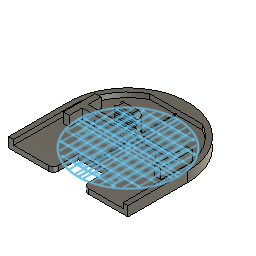
shadowmask_wafer_cleaver (Autodesk Fusion 360 design; units mm, degrees)
Autodesk Fusion 360 part; units mm, degrees
note: some values were not read from the file. Set by a fixed rule: which sketch regions a step uses.
(part 1 of 3)
sketch "wafer_condensed" plane through (0, 0, 0) normal (0, 0, 1) x (1, 0, 0)
  line L0 (3.9115, 15.9115) -> (2, 15.9115)
  line L1 (-4.0885, 2) -> (-4.0885, 3.9115)
  line L2 (-38.9115, 4.0885) -> (-39.0885, 4.0885)
  line L3 (-24.9115, 3.9115) -> (-18.0885, 3.9115)
  line L4 (-31.9115, 3.9115) -> (-25.0885, 3.9115)
  line L5 (-11.0885, 3.9115) -> (-10.9115, 3.9115)
  line L6 (-25.0885, 4.0885) -> (-25.0885, 3.9115)
  line L7 (-39.0885, 3.9115) -> (-38.9115, 3.9115)
  line L8 (-25.0885, 3.9115) -> (-31.9115, 3.9115)
  line L9 (-3.9115, 3.9115) -> (-2, 3.9115)
  line L10 (-32.0885, 3.9115) -> (-31.9115, 3.9115)
  line L11 (-10.9115, 3.9115) -> (-4.0885, 3.9115)
  line L12 (-25.0885, 3.9115) -> (-24.9115, 3.9115)
  line L13 (-31.9115, 3.9115) -> (-31.9115, 4.0885)
  line L14 (-4.0885, 3.9115) -> (-3.9115, 3.9115)
  line L15 (-3.9115, 3.9115) -> (-3.9115, 2)
  line L16 (-2, 3.9115) -> (-3.9115, 3.9115)
  line L17 (-32.0885, 3.9115) -> (-38.9115, 3.9115)
  line L18 (-32.0885, 4.0885) -> (-32.0885, 3.9115)
  line L19 (-10.9115, 3.9115) -> (-10.9115, 2)
  line L20 (-24.9115, 3.9115) -> (-24.9115, 4.0885)
  line L21 (-4.0885, 3.9115) -> (-10.9115, 3.9115)
  line L22 (-18.0885, 3.9115) -> (-17.9115, 3.9115)
  line L23 (-10.9115, 2) -> (-11.0885, 2)
  line L24 (-17.9115, 3.9115) -> (-11.0885, 3.9115)
  line L25 (-38.9115, 3.9115) -> (-38.9115, 4.0885)
  line L26 (-24.9115, 4.0885) -> (-25.0885, 4.0885)
  line L27 (-3.9115, 2) -> (-4.0885, 2)
  line L28 (-11.0885, 2) -> (-11.0885, 3.9115)
  line L29 (-39.0885, 4.0885) -> (-39.0885, 3.9115)
  line L30 (-18.0885, 3.9115) -> (-24.9115, 3.9115)
  line L31 (-38.9115, 3.9115) -> (-32.0885, 3.9115)
  line L32 (-45.9115, 2) -> (-46.0885, 2)
  line L33 (-25.0885, 3.9115) -> (-31.9115, 3.9115)
  line L34 (-45.9115, 3.9115) -> (-45.9115, 2)
  line L35 (-39.0885, 3.9115) -> (-45.9115, 3.9115)
  line L36 (-32.0885, 2) -> (-32.0885, 3.9115)
  line L37 (-18.0885, 2) -> (-18.0885, 3.9115)
  line L38 (-18.0885, 3.9115) -> (-24.9115, 3.9115)
  line L39 (-39.0885, 2) -> (-39.0885, 3.9115)
  line L40 (-38.9115, 2) -> (-39.0885, 2)
  line L41 (-31.9115, 2) -> (-32.0885, 2)
  line L42 (-10.9115, -46.7226) -> (-11.0885, -46.7226)
  line L43 (-24.9115, 3.9115) -> (-24.9115, 2)
  line L44 (-11.0885, -46.7226) -> (-11.0885, -40.0885)
  line L45 (-32.0885, 3.9115) -> (-38.9115, 3.9115)
  line L46 (-17.9115, 2) -> (-18.0885, 2)
  line L47 (-11.0885, -40.0885) -> (-17.9115, -40.0885)
  line L48 (-4.0885, -47.833) -> (-4.0885, -40.0885)
  line L49 (-24.9115, 2) -> (-25.0885, 2)
  line L50 (-17.9115, 3.9115) -> (-17.9115, 2)
  line L51 (-11.0885, 3.9115) -> (-17.9115, 3.9115)
  line L52 (-10.9115, -40.0885) -> (-10.9115, -46.7226)
  line L53 (-25.0885, 2) -> (-25.0885, 3.9115)
  line L54 (-4.0885, -40.0885) -> (-10.9115, -40.0885)
  line L55 (-31.9115, 3.9115) -> (-31.9115, 2)
  line L56 (-38.9115, 3.9115) -> (-38.9115, 2)
  line L57 (-17.9115, 39.9115) -> (-17.9115, 28.0885)
  line L58 (-11.0885, 27.9115) -> (-17.9115, 27.9115)
  line L59 (-3.9115, 28.0885) -> (-4.0885, 28.0885)
  line L60 (-24.9115, 39.9115) -> (-24.9115, 28.0885)
  line L61 (-38.9115, 27.9115) -> (-38.9115, 16.0885)
  line L62 (-4.0885, 16.0885) -> (-4.0885, 27.9115)
  line L63 (-17.9115, 16.0885) -> (-11.0885, 16.0885)
  line L64 (-18.0885, 28.0885) -> (-18.0885, 39.9115)
  line L65 (-18.0885, 16.0885) -> (-18.0885, 27.9115)
  line L66 (-38.9872, 27.9821) -> (-38.9872, 27.9115)
  line L67 (-17.9115, 16.0885) -> (-18.0885, 16.0885)
  line L68 (-32.0885, 16.0885) -> (-31.9115, 16.0885)
  line L69 (-32.0885, 16.0885) -> (-32.0885, 27.9115)
  line L70 (-18.0885, 27.9115) -> (-17.9115, 27.9115)
  line L71 (-31.9115, 16.0885) -> (-32.0885, 16.0885)
  line L72 (-32.0885, 28.0885) -> (-32.0885, 27.9115)
  line L73 (-3.9115, 16.0885) -> (-4.0885, 16.0885)
  line L74 (-25.0885, 16.0885) -> (-25.0885, 27.9115)
  line L75 (-11.0885, 28.0885) -> (-11.0885, 27.9115)
  line L76 (-31.9115, 27.9115) -> (-31.9115, 16.0885)
  line L77 (-11.0885, 15.9115) -> (-17.9115, 15.9115)
  line L78 (-10.9115, 15.9115) -> (-10.9115, 16.0885)
  line L79 (-25.0885, 28.0885) -> (-25.0885, 27.9115)
  line L80 (-2, 27.9115) -> (-3.9115, 27.9115)
  line L81 (-24.9115, 16.0885) -> (-25.0885, 16.0885)
  line L82 (-11.0885, 15.9115) -> (-10.9115, 15.9115)
  line L83 (-17.9115, 28.0885) -> (-18.0885, 28.0885)
  line L84 (-3.9115, 27.9115) -> (-2, 27.9115)
  line L85 (-10.9115, 27.9115) -> (-4.0885, 27.9115)
  line L86 (-10.9115, 28.0885) -> (-4.0885, 28.0885)
  line L87 (-25.0885, 27.9115) -> (-31.9115, 27.9115)
  line L88 (-25.0885, 15.9115) -> (-24.9115, 15.9115)
  line L89 (-2, 16.0885) -> (-2, 15.9115)
  line L90 (-31.9115, 27.9115) -> (-31.9115, 28.0885)
  line L91 (-11.0885, 27.9115) -> (-17.9115, 27.9115)
  line L92 (-18.0885, 28.0885) -> (-17.9115, 28.0885)
  line L93 (-17.9115, 27.9115) -> (-17.9115, 28.0885)
  line L94 (-24.9115, 28.0885) -> (-18.0885, 28.0885)
  line L95 (-4.0885, 27.9115) -> (-10.9115, 27.9115)
  line L96 (-4.0885, 4.0885) -> (-3.9115, 4.0885)
  line L97 (-10.9115, 28.0885) -> (-11.0885, 28.0885)
  line L98 (-17.9115, 28.0885) -> (-18.0885, 28.0885)
  line L99 (-25.0885, 4.0885) -> (-24.9115, 4.0885)
  line L100 (-31.9115, 15.9115) -> (-31.9115, 16.0885)
  line L101 (-25.0885, 15.9115) -> (-31.9115, 15.9115)
  line L102 (-24.9115, 15.9115) -> (-18.0885, 15.9115)
  line L103 (-31.9115, 28.0885) -> (-32.0885, 28.0885)
  line L104 (-4.0885, 16.0885) -> (-4.0885, 15.9115)
  line L105 (-11.0885, 4.0885) -> (-10.9115, 4.0885)
  line L106 (-18.0885, 16.0885) -> (-17.9115, 16.0885)
  line L107 (-25.0885, 4.0885) -> (-25.0885, 15.9115)
  line L108 (-4.0885, 27.9115) -> (-3.9115, 27.9115)
  line L109 (-17.9115, 27.9115) -> (-11.0885, 27.9115)
  line L110 (-25.0885, 27.9115) -> (-31.9115, 27.9115)
  line L111 (-11.0885, 16.0885) -> (-11.0885, 27.9115)
  line L112 (-17.9115, 15.9115) -> (-17.9115, 16.0885)
  line L113 (-4.0885, 27.9115) -> (-10.9115, 27.9115)
  line L114 (-11.0885, 27.9115) -> (-10.9115, 27.9115)
  line L115 (-32.0885, 4.0885) -> (-31.9115, 4.0885)
  line L116 (-18.0885, 27.9115) -> (-24.9115, 27.9115)
  line L117 (-4.0885, 28.0885) -> (-4.0885, 27.9115)
  line L118 (-24.9115, 4.0885) -> (-18.0885, 4.0885)
  line L119 (-11.0885, 28.0885) -> (-10.9115, 28.0885)
  line L120 (-2, 4.0885) -> (-2, 3.9115)
  line L121 (-2, 15.9115) -> (-3.9115, 15.9115)
  line L122 (-11.0885, 16.0885) -> (-10.9115, 16.0885)
  line L123 (-10.9115, 27.9115) -> (-10.9115, 28.0885)
  line L124 (-4.0885, 4.0885) -> (-4.0885, 15.9115)
  line L125 (-18.0885, 28.0885) -> (-18.0885, 27.9115)
  line L126 (-4.0885, 15.9115) -> (-10.9115, 15.9115)
  line L127 (-2, 15.9115) -> (-3.9115, 15.9115)
  line L128 (-18.0885, 4.0885) -> (-18.0885, 15.9115)
  line L129 (-17.9115, 15.9115) -> (-17.9115, 4.0885)
  line L130 (-17.9115, 4.0885) -> (-11.0885, 4.0885)
  line L131 (-11.0885, 15.9115) -> (-17.9115, 15.9115)
  line L132 (-4.0885, 15.9115) -> (-10.9115, 15.9115)
  line L133 (-3.9115, 4.0885) -> (-2, 4.0885)
  line L134 (-10.9115, 4.0885) -> (-11.0885, 4.0885)
  line L135 (-3.9115, 15.9115) -> (-3.9115, 4.0885)
  line L136 (-25.0885, 16.0885) -> (-24.9115, 16.0885)
  line L137 (-25.0885, 15.9115) -> (-31.9115, 15.9115)
  line L138 (-18.0885, 15.9115) -> (-24.9115, 15.9115)
  line L139 (-38.9115, 27.9821) -> (-38.9872, 27.9821)
  line L140 (-3.9115, 15.9115) -> (-2, 15.9115)
  line L141 (-17.9115, 28.0885) -> (-11.0885, 28.0885)
  line L142 (-4.0885, 15.9115) -> (-3.9115, 15.9115)
  line L143 (-24.9115, 15.9115) -> (-24.9115, 4.0885)
  line L144 (-24.9115, 16.0885) -> (-18.0885, 16.0885)
  line L145 (-3.9115, 16.0885) -> (-2, 16.0885)
  line L146 (-17.9115, 27.9115) -> (-17.9115, 16.0885)
  line L147 (-18.0885, 4.0885) -> (-17.9115, 4.0885)
  line L148 (-4.0885, 16.0885) -> (-3.9115, 16.0885)
  line L149 (-10.9115, 16.0885) -> (-4.0885, 16.0885)
  line L150 (-24.9115, 16.0885) -> (-25.0885, 16.0885)
  line L151 (-32.0885, 27.9115) -> (-31.9115, 27.9115)
  line L152 (-10.9115, 15.9115) -> (-4.0885, 15.9115)
  line L153 (-10.9115, 15.9115) -> (-10.9115, 4.0885)
  line L154 (-32.0885, 4.0885) -> (-32.0885, 15.9115)
  line L155 (-3.9115, 27.9115) -> (-3.9115, 16.0885)
  line L156 (-25.0885, 16.0885) -> (-25.0885, 15.9115)
  line L157 (-32.0885, 15.9115) -> (-31.9115, 15.9115)
  line L158 (-32.0885, 27.9115) -> (-38.9115, 27.9115)
  line L159 (-31.9115, 16.0885) -> (-25.0885, 16.0885)
  line L160 (-32.0885, 15.9115) -> (-38.9115, 15.9115)
  line L161 (-31.9115, 16.0885) -> (-32.0885, 16.0885)
  line L162 (-38.9115, 27.9115) -> (-38.9115, 27.9821)
  line L163 (-18.0885, 27.9115) -> (-24.9115, 27.9115)
  line L164 (-24.9115, 27.9115) -> (-24.9115, 28.0885)
  line L165 (-18.0885, 39.9115) -> (-24.9115, 39.9115)
  line L166 (-4.0885, 28.0885) -> (-3.9115, 28.0885)
  line L167 (-17.9115, 16.0885) -> (-18.0885, 16.0885)
  line L168 (-24.9115, 15.9115) -> (-24.9115, 16.0885)
  line L169 (-24.9115, 27.9115) -> (-18.0885, 27.9115)
  line L170 (-10.9115, 16.0885) -> (-11.0885, 16.0885)
  line L171 (-31.9115, 4.0885) -> (-32.0885, 4.0885)
  line L172 (-2, 28.0885) -> (-2, 27.9115)
  line L173 (-10.9115, 4.0885) -> (-4.0885, 4.0885)
  line L174 (-2, 27.9115) -> (-3.9115, 27.9115)
  line L175 (-24.9115, 28.0885) -> (-25.0885, 28.0885)
  line L176 (-32.0885, 27.9115) -> (-38.9115, 27.9115)
  line L177 (-11.0885, 16.0885) -> (-11.0885, 15.9115)
  line L178 (-3.9115, 4.0885) -> (-4.0885, 4.0885)
  line L179 (-32.0885, 16.0885) -> (-32.0885, 15.9115)
  line L180 (-17.9115, 4.0885) -> (-18.0885, 4.0885)
  line L181 (-31.9115, 4.0885) -> (-25.0885, 4.0885)
  line L182 (-25.0885, 27.9115) -> (-24.9115, 27.9115)
  line L183 (-3.9115, 16.0885) -> (-4.0885, 16.0885)
  line L184 (-38.9115, 15.9115) -> (-38.9115, 4.0885)
  line L185 (-24.9115, 27.9115) -> (-24.9115, 16.0885)
  line L186 (-3.9115, 15.9115) -> (-3.9115, 16.0885)
  line L187 (-31.9115, 15.9115) -> (-31.9115, 4.0885)
  line L188 (-10.9115, 16.0885) -> (-11.0885, 16.0885)
  line L189 (-10.9115, 27.9115) -> (-10.9115, 16.0885)
  line L190 (-31.9115, 15.9115) -> (-25.0885, 15.9115)
  line L191 (-38.9115, 16.0885) -> (-32.0885, 16.0885)
  line L192 (-3.9115, 27.9115) -> (-3.9115, 28.0885)
  line L193 (-18.0885, 15.9115) -> (-17.9115, 15.9115)
  line L194 (-31.9115, 27.9115) -> (-25.0885, 27.9115)
  line L195 (-3.9115, 28.0885) -> (-2, 28.0885)
  line L196 (-18.0885, 15.9115) -> (-24.9115, 15.9115)
  line L197 (-24.9115, 4.0885) -> (-25.0885, 4.0885)
  line L198 (-38.9872, 27.9115) -> (-38.9115, 27.9115)
  line L199 (-11.0885, 4.0885) -> (-11.0885, 15.9115)
  line L200 (-38.9115, 4.0885) -> (-32.0885, 4.0885)
  line L201 (-18.0885, 16.0885) -> (-18.0885, 15.9115)
  line L202 (-17.9115, 15.9115) -> (-11.0885, 15.9115)
  line L203 (-38.9115, 27.9115) -> (-32.0885, 27.9115)
  line L204 (-17.9115, 3.9115) -> (-17.9115, 4.0885)
  line L205 (-4.0885, 4.0885) -> (-4.0885, 3.9115)
  line L206 (-3.9115, 4.0885) -> (-4.0885, 4.0885)
  line L207 (-17.9115, 4.0885) -> (-18.0885, 4.0885)
  line L208 (-11.0885, 3.9115) -> (-17.9115, 3.9115)
  line L209 (-3.9115, 3.9115) -> (-3.9115, 4.0885)
  line L210 (-18.0885, 4.0885) -> (-18.0885, 3.9115)
  line L211 (-2, 3.9115) -> (-3.9115, 3.9115)
  line L212 (-11.0885, 4.0885) -> (-11.0885, 3.9115)
  line L213 (-4.0885, 3.9115) -> (-10.9115, 3.9115)
  line L214 (-10.9115, 3.9115) -> (-10.9115, 4.0885)
  line L215 (-10.9115, 4.0885) -> (-11.0885, 4.0885)
  line L216 (-10.9115, 39.9115) -> (-4.0885, 39.9115)
  line L217 (-11.0885, 28.0885) -> (-11.0885, 39.9115)
  line L218 (-10.9115, 39.9115) -> (-10.9115, 28.0885)
  line L219 (-4.0885, 39.9115) -> (-10.9115, 39.9115)
  line L220 (-3.9115, 28.0885) -> (-4.0885, 28.0885)
  line L221 (-10.9115, 28.0885) -> (-11.0885, 28.0885)
  line L222 (-4.0885, 28.0885) -> (-4.0885, 39.9115)
  line L223 (-11.0885, 39.9115) -> (-17.9115, 39.9115)
  line L224 (-3.9115, 39.9115) -> (-2, 39.9115)
  line L225 (-2, 39.9115) -> (-3.9115, 39.9115)
  line L226 (-4.0885, 39.9115) -> (-3.9115, 39.9115)
  line L227 (-3.9115, 39.9115) -> (-3.9115, 28.0885)
  line L228 (18.0885, 2) -> (17.9115, 2)
  line L229 (3.9115, 40.0885) -> (3.9115, 39.9115)
  line L230 (-46.0885, 3.9115) -> (-47.833, 3.9115)
  line L231 (17.9115, 3.9115) -> (11.0885, 3.9115)
  line L232 (39.0885, 15.9115) -> (39.0885, 16.0885)
  line L233 (18.0885, 40.0885) -> (24.9115, 40.0885)
  line L234 (24.9115, 39.9115) -> (25.0885, 39.9115)
  line L235 (3.9115, 39.9115) -> (2, 39.9115)
  line L236 (-45.9115, 13.7113) -> (-45.9115, 4.0885)
  line L237 (31.9115, 3.9115) -> (25.0885, 3.9115)
  line L238 (46.0885, 3.9115) -> (46.0885, 4.0885)
  line L239 (-25.0885, 39.9115) -> (-26.533, 39.9115)
  line L240 (25.0885, 3.9115) -> (25.0885, 2)
  line L241 (38.9115, 3.9115) -> (32.0885, 3.9115)
  line L242 (38.9115, 2) -> (38.9115, 3.9115)
  line L243 (-25.0885, 40.0885) -> (-25.0885, 39.9115)
  line L244 (46.0885, 4.0885) -> (45.9115, 4.0885)
  line L245 (31.9115, 35.7771) -> (32.0885, 35.7771)
  line L246 (-39.0885, 16.0885) -> (-39.0885, 27.9821)
  line L247 (4.0885, 40.0885) -> (10.9115, 40.0885)
  line L248 (-38.9115, 15.9115) -> (-38.9115, 16.0885)
  line L249 (17.9115, 2) -> (17.9115, 3.9115)
  line L250 (2, 39.9115) -> (2, 40.0885)
  line L251 (2, 40.0885) -> (3.9115, 40.0885)
  line L252 (-24.9115, 39.9115) -> (-24.9115, 40.0885)
  line L253 (38.9872, 27.9821) -> (39.0885, 27.9821)
  line L254 (24.9115, 40.0885) -> (24.9115, 40.9756)
  line L255 (-46.0885, 4.0885) -> (-46.0885, 3.9115)
  line L256 (39.0885, 27.9821) -> (39.0885, 16.0885)
  line L257 (-38.9872, 28.0885) -> (-32.0885, 28.0885)
  line L258 (11.0885, 3.9115) -> (11.0885, 2)
  line L259 (4.0885, 40.0885) -> (3.9115, 40.0885)
  line L260 (4.0885, 39.9115) -> (4.0885, 40.0885)
  line L261 (45.9115, 2) -> (45.9115, 3.9115)
  line L262 (-46.0885, 3.9115) -> (-45.9115, 3.9115)
  line L263 (25.0885, 40.0885) -> (26.533, 40.0885)
  line L264 (-39.0885, 4.0885) -> (-39.0885, 15.9115)
  line L265 (38.9872, 28.0885) -> (38.9872, 27.9821)
  line L266 (47.833, 3.9115) -> (46.0885, 3.9115)
  line L267 (32.0885, 3.9115) -> (32.0885, 2)
  line L268 (11.0885, 46.7226) -> (11.0885, 40.0885)
  line L269 (17.9115, 44.4972) -> (18.0885, 44.4972)
  line L270 (-46.0885, 2) -> (-46.0885, 3.9115)
  line L271 (4.0885, 3.9115) -> (4.0885, 2)
  line L272 (31.9115, 28.0885) -> (31.9115, 35.7771)
  line L273 (10.9115, 39.9115) -> (4.0885, 39.9115)
  line L274 (-45.2548, 15.9115) -> (-45.2548, 16.0885)
  line L275 (24.9115, 3.9115) -> (18.0885, 3.9115)
  line L276 (-39.0885, 15.9115) -> (-45.2548, 15.9115)
  line L277 (-47.833, 3.9115) -> (-47.833, 4.0885)
  line L278 (-45.9115, 4.0885) -> (-46.0885, 4.0885)
  line L279 (10.9115, 3.9115) -> (4.0885, 3.9115)
  line L280 (26.533, 40.0885) -> (26.533, 39.9115)
  line L281 (31.9115, 2) -> (31.9115, 3.9115)
  line L282 (-25.0885, 28.0885) -> (-25.0885, 39.9115)
  line L283 (26.533, 39.9115) -> (25.0885, 39.9115)
  line L284 (-39.0885, 15.9115) -> (-38.9115, 15.9115)
  line L285 (25.0885, 40.9756) -> (25.0885, 40.0885)
  line L286 (32.0885, 2) -> (31.9115, 2)
  line L287 (45.9115, 3.9115) -> (39.0885, 3.9115)
  line L288 (11.0885, 2) -> (10.9115, 2)
  line L289 (25.0885, 39.9115) -> (25.0885, 28.0885)
  line L290 (39.0885, 4.0885) -> (45.9115, 4.0885)
  line L291 (25.0885, 40.0885) -> (24.9115, 40.0885)
  line L292 (-24.9115, 40.0885) -> (-25.0885, 40.0885)
  line L293 (18.0885, 3.9115) -> (18.0885, 2)
  line L294 (4.0885, 2) -> (3.9115, 2)
  line L295 (32.0885, 28.0885) -> (38.9872, 28.0885)
  line L296 (45.9115, 13.7113) -> (46.0885, 13.7113)
  line L297 (32.0885, 35.7771) -> (32.0885, 28.0885)
  line L298 (3.9115, 40.0885) -> (3.9115, 47.833)
  line L299 (24.9115, 2) -> (24.9115, 3.9115)
  line L300 (-47.833, 4.0885) -> (-46.0885, 4.0885)
  line L301 (39.0885, 15.9115) -> (39.0885, 4.0885)
  line L302 (46.0885, 2) -> (45.9115, 2)
  line L303 (45.9115, 4.0885) -> (45.9115, 13.7113)
  line L304 (38.9115, 15.9115) -> (39.0885, 15.9115)
  line L305 (39.0885, 2) -> (38.9115, 2)
  line L306 (3.9115, 47.833) -> (4.0885, 47.833)
  line L307 (46.0885, 3.9115) -> (46.0885, 2)
  line L308 (-39.0885, 16.0885) -> (-39.0885, 15.9115)
  line L309 (47.833, 4.0885) -> (47.833, 3.9115)
  line L310 (25.0885, 2) -> (24.9115, 2)
  line L311 (10.9115, 2) -> (10.9115, 3.9115)
  line L312 (11.0885, 40.0885) -> (17.9115, 40.0885)
  line L313 (-45.9115, 4.0885) -> (-39.0885, 4.0885)
  line L314 (45.2548, 16.0885) -> (45.2548, 15.9115)
  line L315 (-32.0885, 35.7771) -> (-31.9115, 35.7771)
  line L316 (25.0885, 39.9115) -> (25.0885, 40.0885)
  line L317 (46.0885, 13.7113) -> (46.0885, 4.0885)
  line L318 (10.9115, 46.7226) -> (11.0885, 46.7226)
  line L319 (24.9115, 40.9756) -> (25.0885, 40.9756)
  line L320 (18.0885, 44.4972) -> (18.0885, 40.0885)
  line L321 (-25.0885, 39.9115) -> (-24.9115, 39.9115)
  line L322 (-31.9115, 35.7771) -> (-31.9115, 28.0885)
  line L323 (39.0885, 3.9115) -> (39.0885, 2)
  line L324 (-46.0885, 4.0885) -> (-46.0885, 13.7113)
  line L325 (-46.0885, 13.7113) -> (-45.9115, 13.7113)
  line L326 (24.9115, 40.0885) -> (24.9115, 39.9115)
  line L327 (45.9115, 3.9115) -> (46.0885, 3.9115)
  line L328 (25.0885, 28.0885) -> (31.9115, 28.0885)
  line L329 (45.9115, 4.0885) -> (45.9115, 3.9115)
  line L330 (39.0885, 16.0885) -> (45.2548, 16.0885)
  line L331 (38.9115, 16.0885) -> (38.9115, 15.9115)
  line L332 (10.9115, 40.0885) -> (10.9115, 39.9115)
  line L333 (-32.0885, 28.0885) -> (-32.0885, 35.7771)
  line L334 (-39.0885, 27.9821) -> (-38.9872, 27.9821)
  line L335 (10.9115, 40.0885) -> (10.9115, 46.7226)
  line L336 (-45.9115, 3.9115) -> (-45.9115, 4.0885)
  line L337 (-45.2548, 16.0885) -> (-39.0885, 16.0885)
  line L338 (46.0885, 4.0885) -> (47.833, 4.0885)
  line L339 (17.9115, 40.0885) -> (17.9115, 44.4972)
  line L340 (-38.9872, 27.9821) -> (-38.9872, 28.0885)
  line L341 (-31.9115, 28.0885) -> (-25.0885, 28.0885)
  line L342 (45.2548, 15.9115) -> (39.0885, 15.9115)
  line L343 (39.0885, 16.0885) -> (38.9115, 16.0885)
  line L344 (4.0885, 47.833) -> (4.0885, 40.0885)
  line L345 (-38.9115, 16.0885) -> (-39.0885, 16.0885)
  line L346 (-17.9115, 39.9115) -> (-17.9115, 40.0885)
  line L347 (-18.0885, 44.4972) -> (-17.9115, 44.4972)
  line L348 (-25.0885, 40.9756) -> (-24.9115, 40.9756)
  line L349 (-11.0885, 40.0885) -> (-11.0885, 46.7226)
  line L350 (-18.0885, 40.0885) -> (-18.0885, 39.9115)
  line L351 (-11.0885, 39.9115) -> (-17.9115, 39.9115)
  line L352 (-11.0885, 40.0885) -> (-11.0885, 39.9115)
  line L353 (-18.0885, 39.9115) -> (-17.9115, 39.9115)
  line L354 (-26.533, 39.9115) -> (-26.533, 40.0885)
  line L355 (-26.533, 40.0885) -> (-25.0885, 40.0885)
  line L356 (-4.0885, 40.0885) -> (-4.0885, 47.833)
  line L357 (-3.9115, 39.9115) -> (-3.9115, 40.0885)
  line L358 (-24.9115, 40.0885) -> (-18.0885, 40.0885)
  line L359 (-3.9115, 40.0885) -> (-4.0885, 40.0885)
  line L360 (-17.9115, 40.0885) -> (-18.0885, 40.0885)
  line L361 (-17.9115, 40.0885) -> (-11.0885, 40.0885)
  line L362 (-4.0885, 47.833) -> (-3.9115, 47.833)
  line L363 (-10.9115, 40.0885) -> (-4.0885, 40.0885)
  line L364 (-3.9115, 40.0885) -> (-2, 40.0885)
  line L365 (-17.9115, 44.4972) -> (-17.9115, 40.0885)
  line L366 (-25.0885, 40.0885) -> (-25.0885, 40.9756)
  line L367 (-11.0885, 46.7226) -> (-10.9115, 46.7226)
  line L368 (-2, 40.0885) -> (-2, 39.9115)
  line L369 (-10.9115, 46.7226) -> (-10.9115, 40.0885)
  line L370 (-4.0885, 40.0885) -> (-4.0885, 39.9115)
  line L371 (-24.9115, 40.9756) -> (-24.9115, 40.0885)
  line L372 (-2, 39.9115) -> (-3.9115, 39.9115)
  line L373 (-10.9115, 40.0885) -> (-11.0885, 40.0885)
  line L374 (-4.0885, 39.9115) -> (-10.9115, 39.9115)
  line L375 (-18.0885, 40.0885) -> (-18.0885, 44.4972)
  line L376 (-10.9115, 39.9115) -> (-10.9115, 40.0885)
  line L377 (-3.9115, 47.833) -> (-3.9115, 40.0885)
  line L378 (-11.0885, 39.9115) -> (-10.9115, 39.9115)
  line L379 (-17.9115, 39.9115) -> (-11.0885, 39.9115)
  line L380 (10.9115, -15.9115) -> (4.0885, -15.9115)
  line L381 (4.0885, 4.0885) -> (3.9115, 4.0885)
  line L382 (47.833, -3.9115) -> (47.833, -4.0885)
  line L383 (47.833, -4.0885) -> (46.0885, -4.0885)
  line L384 (4.0885, 3.9115) -> (10.9115, 3.9115)
  line L385 (10.9115, 3.9115) -> (11.0885, 3.9115)
  line L386 (17.9115, 3.9115) -> (18.0885, 3.9115)
  line L387 (18.0885, 4.0885) -> (17.9115, 4.0885)
  line L388 (4.0885, -15.9115) -> (3.9115, -15.9115)
  line L389 (11.0885, 3.9115) -> (17.9115, 3.9115)
  line L390 (4.0885, -15.9115) -> (10.9115, -15.9115)
  line L391 (24.9115, -40.9756) -> (24.9115, -40.0885)
  line L392 (38.9115, -16.0885) -> (39.0885, -16.0885)
  line L393 (32.0885, 4.0885) -> (31.9115, 4.0885)
  line L394 (11.0885, 4.0885) -> (17.9115, 4.0885)
  line L395 (18.0885, -15.9115) -> (17.9115, -15.9115)
  line L396 (25.0885, 4.0885) -> (31.9115, 4.0885)
  line L397 (3.9115, 4.0885) -> (4.0885, 4.0885)
  line L398 (11.0885, -40.0885) -> (11.0885, -46.7226)
  line L399 (26.533, -39.9115) -> (26.533, -40.0885)
  line L400 (25.0885, -39.9115) -> (26.533, -39.9115)
  line L401 (11.0885, -46.7226) -> (10.9115, -46.7226)
  line L402 (39.0885, -15.9115) -> (45.2548, -15.9115)
  line L403 (45.2548, -15.9115) -> (45.2548, -16.0885)
  line L404 (45.9115, -4.0885) -> (39.0885, -4.0885)
  line L405 (39.0885, -16.0885) -> (39.0885, -27.9821)
  line L406 (4.0885, -40.0885) -> (4.0885, -47.833)
  line L407 (45.2548, -16.0885) -> (39.0885, -16.0885)
  line L408 (38.9115, 3.9115) -> (39.0885, 3.9115)
  line L409 (39.0885, -15.9115) -> (38.9115, -15.9115)
  line L410 (32.0885, -35.7771) -> (31.9115, -35.7771)
  line L411 (10.9115, -40.0885) -> (4.0885, -40.0885)
  line L412 (24.9115, 3.9115) -> (25.0885, 3.9115)
  line L413 (10.9115, -46.7226) -> (10.9115, -40.0885)
  line L414 (38.9872, -28.0885) -> (32.0885, -28.0885)
  line L415 (25.0885, -28.0885) -> (25.0885, -39.9115)
  line L416 (31.9115, -28.0885) -> (25.0885, -28.0885)
  line L417 (32.0885, -28.0885) -> (32.0885, -35.7771)
  line L418 (18.0885, 15.9115) -> (18.0885, 4.0885)
  line L419 (32.0885, 15.9115) -> (32.0885, 4.0885)
  line L420 (25.0885, -40.0885) -> (25.0885, -39.9115)
  line L421 (3.9115, 3.9115) -> (2, 3.9115)
  line L422 (18.0885, 3.9115) -> (24.9115, 3.9115)
  line L423 (18.0885, -44.4972) -> (17.9115, -44.4972)
  line L424 (25.0885, 3.9115) -> (31.9115, 3.9115)
  line L425 (4.0885, -47.833) -> (3.9115, -47.833)
  line L426 (38.9115, 15.9115) -> (32.0885, 15.9115)
  line L427 (39.0885, -4.0885) -> (39.0885, -15.9115)
  line L428 (32.0885, 3.9115) -> (38.9115, 3.9115)
  line L429 (10.9115, 4.0885) -> (10.9115, 15.9115)
  line L430 (32.0885, -15.9115) -> (31.9115, -15.9115)
  line L431 (3.9115, 2) -> (3.9115, 3.9115)
  line L432 (10.9115, -15.9115) -> (10.9115, -4.0885)
  line L433 (3.9115, 3.9115) -> (4.0885, 3.9115)
  line L434 (24.9115, 15.9115) -> (18.0885, 15.9115)
  line L435 (25.0885, -40.0885) -> (25.0885, -40.9756)
  line L436 (10.9115, 15.9115) -> (4.0885, 15.9115)
  line L437 (11.0885, -15.9115) -> (10.9115, -15.9115)
  line L438 (45.9115, -3.9115) -> (45.9115, -4.0885)
  line L439 (11.0885, -15.9115) -> (17.9115, -15.9115)
  line L440 (46.0885, -4.0885) -> (46.0885, -13.7113)
  line L441 (17.9115, -4.0885) -> (18.0885, -4.0885)
  line L442 (3.9115, -15.9115) -> (2, -15.9115)
  line L443 (3.9115, 4.0885) -> (3.9115, 3.9115)
  line L444 (25.0885, 4.0885) -> (24.9115, 4.0885)
  line L445 (25.0885, -15.9115) -> (31.9115, -15.9115)
  line L446 (10.9115, -4.0885) -> (11.0885, -4.0885)
  line L447 (17.9115, -15.9115) -> (11.0885, -15.9115)
  line L448 (31.9115, 3.9115) -> (32.0885, 3.9115)
  line L449 (39.0885, 3.9115) -> (39.0885, 4.0885)
  line L450 (18.0885, -4.0885) -> (18.0885, -15.9115)
  line L451 (31.9115, -15.9115) -> (31.9115, -16.0885)
  line L452 (4.0885, 3.9115) -> (4.0885, 4.0885)
  line L453 (45.9115, -4.0885) -> (46.0885, -4.0885)
  line L454 (11.0885, 4.0885) -> (10.9115, 4.0885)
  line L455 (46.0885, -4.0885) -> (46.0885, -3.9115)
  line L456 (11.0885, 15.9115) -> (11.0885, 4.0885)
  line L457 (24.9115, -15.9115) -> (18.0885, -15.9115)
  line L458 (17.9115, -15.9115) -> (17.9115, -4.0885)
  line L459 (3.9115, 3.9115) -> (2, 3.9115)
  line L460 (3.9115, -15.9115) -> (3.9115, -4.0885)
  line L461 (24.9115, 4.0885) -> (25.0885, 4.0885)
  line L462 (2, 3.9115) -> (2, 4.0885)
  line L463 (2, -15.9115) -> (3.9115, -15.9115)
  line L464 (11.0885, -4.0885) -> (11.0885, -15.9115)
  line L465 (4.0885, -4.0885) -> (4.0885, -15.9115)
  line L466 (38.9115, 4.0885) -> (38.9115, 3.9115)
  line L467 (32.0885, -16.0885) -> (32.0885, -15.9115)
  line L468 (17.9115, 4.0885) -> (17.9115, 15.9115)
  line L469 (31.9115, -15.9115) -> (25.0885, -15.9115)
  line L470 (17.9115, 15.9115) -> (11.0885, 15.9115)
  line L471 (39.0885, 4.0885) -> (38.9115, 4.0885)
  line L472 (31.9115, -16.0885) -> (32.0885, -16.0885)
  line L473 (46.0885, -3.9115) -> (47.833, -3.9115)
  line L474 (25.0885, -15.9115) -> (24.9115, -15.9115)
  line L475 (45.9115, -13.7113) -> (45.9115, -4.0885)
  line L476 (46.0885, -13.7113) -> (45.9115, -13.7113)
  line L477 (17.9115, 4.0885) -> (18.0885, 4.0885)
  line L478 (3.9115, -4.0885) -> (4.0885, -4.0885)
  line L479 (24.9115, 4.0885) -> (24.9115, 15.9115)
  line L480 (31.9115, 15.9115) -> (25.0885, 15.9115)
  line L481 (25.0885, 15.9115) -> (25.0885, 4.0885)
  line L482 (38.9115, 4.0885) -> (38.9115, 15.9115)
  line L483 (10.9115, 4.0885) -> (11.0885, 4.0885)
  line L484 (31.9115, 4.0885) -> (31.9115, 15.9115)
  line L485 (18.0885, 4.0885) -> (24.9115, 4.0885)
  line L486 (17.9115, -40.0885) -> (11.0885, -40.0885)
  line L487 (17.9115, -44.4972) -> (17.9115, -40.0885)
  line L488 (18.0885, -40.0885) -> (18.0885, -44.4972)
  line L489 (24.9115, -40.0885) -> (18.0885, -40.0885)
  line L490 (38.9115, 3.9115) -> (32.0885, 3.9115)
  line L491 (24.9115, -40.0885) -> (25.0885, -40.0885)
  line L492 (2, 4.0885) -> (3.9115, 4.0885)
  line L493 (4.0885, 4.0885) -> (10.9115, 4.0885)
  line L494 (24.9115, -39.9115) -> (24.9115, -40.0885)
  line L495 (25.0885, -39.9115) -> (24.9115, -39.9115)
  line L496 (25.0885, -40.9756) -> (24.9115, -40.9756)
  line L497 (38.9115, -15.9115) -> (38.9115, -16.0885)
  line L498 (31.9115, -35.7771) -> (31.9115, -28.0885)
  line L499 (39.0885, -27.9821) -> (38.9872, -27.9821)
  line L500 (10.9115, 4.0885) -> (10.9115, 3.9115)
  line L501 (10.9115, 3.9115) -> (4.0885, 3.9115)
  line L502 (38.9872, -27.9821) -> (38.9872, -28.0885)
  line L503 (26.533, -40.0885) -> (25.0885, -40.0885)
  line L504 (24.9115, -4.0885) -> (25.0885, -4.0885)
  line L505 (24.9115, -15.9115) -> (24.9115, -4.0885)
  line L506 (18.0885, -15.9115) -> (24.9115, -15.9115)
  line L507 (31.9115, -15.9115) -> (31.9115, -4.0885)
  line L508 (25.0885, -15.9115) -> (31.9115, -15.9115)
  line L509 (25.0885, -4.0885) -> (25.0885, -15.9115)
  line L510 (32.0885, -15.9115) -> (38.9115, -15.9115)
  line L511 (39.0885, -16.0885) -> (39.0885, -15.9115)
  line L512 (2, 3.9115) -> (3.9115, 3.9115)
  line L513 (32.0885, -4.0885) -> (32.0885, -15.9115)
  line L514 (31.9115, -4.0885) -> (32.0885, -4.0885)
  line L515 (32.0885, -4.0885) -> (31.9115, -4.0885)
  line L516 (38.9115, -4.0885) -> (32.0885, -4.0885)
  line L517 (38.9115, -15.9115) -> (38.9115, -4.0885)
  line L518 (24.9115, -4.0885) -> (18.0885, -4.0885)
  line L519 (25.0885, -4.0885) -> (24.9115, -4.0885)
  line L520 (31.9115, -4.0885) -> (25.0885, -4.0885)
  line L521 (11.0885, -4.0885) -> (10.9115, -4.0885)
  line L522 (17.9115, -4.0885) -> (11.0885, -4.0885)
  line L523 (18.0885, -4.0885) -> (17.9115, -4.0885)
  line L524 (3.9115, -4.0885) -> (2, -4.0885)
  line L525 (4.0885, -4.0885) -> (3.9115, -4.0885)
  line L526 (10.9115, -4.0885) -> (4.0885, -4.0885)
  line L527 (17.9115, 3.9115) -> (11.0885, 3.9115)
  line L528 (17.9115, 4.0885) -> (17.9115, 3.9115)
  line L529 (18.0885, 4.0885) -> (17.9115, 4.0885)
  line L530 (11.0885, 4.0885) -> (10.9115, 4.0885)
  line L531 (11.0885, 3.9115) -> (11.0885, 4.0885)
  line L532 (31.9115, 4.0885) -> (31.9115, 3.9115)
  line L533 (32.0885, 4.0885) -> (31.9115, 4.0885)
  line L534 (32.0885, 3.9115) -> (32.0885, 4.0885)
  line L535 (3.9115, -3.9115) -> (3.9115, -4.0885)
  line L536 (2, -3.9115) -> (3.9115, -3.9115)
  line L537 (2, -4.0885) -> (2, -3.9115)
  line L538 (4.0885, -3.9115) -> (10.9115, -3.9115)
  line L539 (4.0885, -4.0885) -> (4.0885, -3.9115)
  line L540 (3.9115, -4.0885) -> (4.0885, -4.0885)
  line L541 (11.0885, -4.0885) -> (11.0885, -3.9115)
  line L542 (10.9115, -4.0885) -> (11.0885, -4.0885)
  line L543 (10.9115, -3.9115) -> (10.9115, -4.0885)
  line L544 (17.9115, -4.0885) -> (18.0885, -4.0885)
  line L545 (17.9115, -3.9115) -> (17.9115, -4.0885)
  line L546 (11.0885, -3.9115) -> (17.9115, -3.9115)
  line L547 (24.9115, -3.9115) -> (24.9115, -4.0885)
  line L548 (18.0885, -3.9115) -> (24.9115, -3.9115)
  line L549 (18.0885, -4.0885) -> (18.0885, -3.9115)
  line L550 (25.0885, -3.9115) -> (31.9115, -3.9115)
  line L551 (25.0885, -4.0885) -> (25.0885, -3.9115)
  line L552 (24.9115, -4.0885) -> (25.0885, -4.0885)
  line L553 (32.0885, -4.0885) -> (32.0885, -3.9115)
  line L554 (31.9115, -4.0885) -> (32.0885, -4.0885)
  line L555 (31.9115, -3.9115) -> (31.9115, -4.0885)
  line L556 (18.0885, 3.9115) -> (18.0885, 4.0885)
  line L557 (24.9115, 3.9115) -> (18.0885, 3.9115)
  line L558 (24.9115, 4.0885) -> (24.9115, 3.9115)
  line L559 (32.0885, 4.0885) -> (38.9115, 4.0885)
  line L560 (38.9115, -4.0885) -> (39.0885, -4.0885)
  line L561 (38.9115, -3.9115) -> (38.9115, -4.0885)
  line L562 (32.0885, -3.9115) -> (38.9115, -3.9115)
  line L563 (38.9115, -3.9115) -> (32.0885, -3.9115)
  line L564 (39.0885, -3.9115) -> (38.9115, -3.9115)
  line L565 (39.0885, -4.0885) -> (39.0885, -3.9115)
  line L566 (25.0885, -3.9115) -> (24.9115, -3.9115)
  line L567 (31.9115, -3.9115) -> (25.0885, -3.9115)
  line L568 (32.0885, -3.9115) -> (31.9115, -3.9115)
  line L569 (17.9115, -3.9115) -> (11.0885, -3.9115)
  line L570 (18.0885, -3.9115) -> (17.9115, -3.9115)
  line L571 (24.9115, -3.9115) -> (18.0885, -3.9115)
  line L572 (4.0885, -3.9115) -> (3.9115, -3.9115)
  line L573 (10.9115, -3.9115) -> (4.0885, -3.9115)
  line L574 (11.0885, -3.9115) -> (10.9115, -3.9115)
  line L575 (3.9115, -3.9115) -> (3.9115, -2)
  line L576 (2, -3.9115) -> (3.9115, -3.9115)
  line L577 (3.9115, -3.9115) -> (2, -3.9115)
  line L578 (4.0885, -3.9115) -> (10.9115, -3.9115)
  line L579 (4.0885, -2) -> (4.0885, -3.9115)
  line L580 (3.9115, -2) -> (4.0885, -2)
  line L581 (11.0885, -2) -> (11.0885, -3.9115)
  line L582 (10.9115, -2) -> (11.0885, -2)
  line L583 (10.9115, -3.9115) -> (10.9115, -2)
  line L584 (25.0885, 4.0885) -> (24.9115, 4.0885)
  line L585 (25.0885, 3.9115) -> (25.0885, 4.0885)
  line L586 (31.9115, 3.9115) -> (25.0885, 3.9115)
  line L587 (31.9115, 4.0885) -> (32.0885, 4.0885)
  line L588 (17.9115, -2) -> (18.0885, -2)
  line L589 (17.9115, -3.9115) -> (17.9115, -2)
  line L590 (11.0885, -3.9115) -> (17.9115, -3.9115)
  line L591 (24.9115, -3.9115) -> (24.9115, -2)
  line L592 (18.0885, -3.9115) -> (24.9115, -3.9115)
  line L593 (18.0885, -2) -> (18.0885, -3.9115)
  line L594 (25.0885, -3.9115) -> (31.9115, -3.9115)
  line L595 (25.0885, -2) -> (25.0885, -3.9115)
  line L596 (24.9115, -2) -> (25.0885, -2)
  line L597 (32.0885, -2) -> (32.0885, -3.9115)
  line L598 (31.9115, -2) -> (32.0885, -2)
  line L599 (31.9115, -3.9115) -> (31.9115, -2)
  line L600 (38.9115, -2) -> (39.0885, -2)
  line L601 (38.9115, -3.9115) -> (38.9115, -2)
  line L602 (32.0885, -3.9115) -> (38.9115, -3.9115)
  line L603 (45.9115, -3.9115) -> (45.9115, -2)
  line L604 (39.0885, -3.9115) -> (45.9115, -3.9115)
  line L605 (39.0885, -2) -> (39.0885, -3.9115)
  line L606 (46.0885, -3.9115) -> (45.9115, -3.9115)
  line L607 (46.0885, -2) -> (46.0885, -3.9115)
  line L608 (45.9115, -2) -> (46.0885, -2)
  line L609 (10.9115, 28.0885) -> (11.0885, 28.0885)
  line L610 (38.9115, 16.0885) -> (38.9115, 27.9115)
  line L611 (25.0885, 16.0885) -> (24.9115, 16.0885)
  line L612 (17.9115, 40.0885) -> (17.9115, 39.9115)
  line L613 (17.9115, 27.9115) -> (11.0885, 27.9115)
  line L614 (38.9115, 27.9821) -> (38.9115, 27.9115)
  line L615 (18.0885, 28.0885) -> (24.9115, 28.0885)
  line L616 (24.9115, 27.9115) -> (18.0885, 27.9115)
  line L617 (2, 39.9115) -> (3.9115, 39.9115)
  line L618 (31.9115, 16.0885) -> (31.9115, 15.9115)
  line L619 (38.9872, 27.9821) -> (38.9115, 27.9821)
  line L620 (32.0885, 16.0885) -> (38.9115, 16.0885)
  line L621 (31.9115, 16.0885) -> (32.0885, 16.0885)
  line L622 (38.9115, 27.9115) -> (32.0885, 27.9115)
  line L623 (38.9115, 27.9115) -> (38.9872, 27.9115)
  line L624 (10.9115, 27.9115) -> (4.0885, 27.9115)
  line L625 (11.0885, 28.0885) -> (17.9115, 28.0885)
  line L626 (32.0885, 27.9115) -> (32.0885, 28.0885)
  line L627 (31.9115, 16.0885) -> (31.9115, 27.9115)
  line L628 (18.0885, 40.0885) -> (17.9115, 40.0885)
  line L629 (38.9872, 27.9115) -> (38.9872, 27.9821)
  line L630 (32.0885, 27.9115) -> (38.9115, 27.9115)
  line L631 (3.9115, 16.0885) -> (3.9115, 27.9115)
  line L632 (4.0885, 27.9115) -> (4.0885, 16.0885)
  line L633 (17.9115, 27.9115) -> (18.0885, 27.9115)
  line L634 (18.0885, 27.9115) -> (24.9115, 27.9115)
  line L635 (17.9115, 16.0885) -> (17.9115, 27.9115)
  line L636 (11.0885, 16.0885) -> (10.9115, 16.0885)
  line L637 (10.9115, 16.0885) -> (10.9115, 27.9115)
  line L638 (11.0885, 27.9115) -> (11.0885, 16.0885)
  line L639 (2, 27.9115) -> (3.9115, 27.9115)
  line L640 (25.0885, 15.9115) -> (25.0885, 16.0885)
  line L641 (31.9115, 15.9115) -> (25.0885, 15.9115)
  line L642 (25.0885, 16.0885) -> (24.9115, 16.0885)
  line L643 (24.9115, 27.9115) -> (25.0885, 27.9115)
  line L644 (24.9115, 16.0885) -> (24.9115, 15.9115)
  line L645 (10.9115, 15.9115) -> (4.0885, 15.9115)
  line L646 (31.9115, 27.9115) -> (32.0885, 27.9115)
  line L647 (4.0885, 16.0885) -> (10.9115, 16.0885)
  line L648 (11.0885, 27.9115) -> (17.9115, 27.9115)
  line L649 (4.0885, 16.0885) -> (3.9115, 16.0885)
  line L650 (3.9115, 39.9115) -> (4.0885, 39.9115)
  line L651 (3.9115, 27.9115) -> (4.0885, 27.9115)
  line L652 (10.9115, 27.9115) -> (11.0885, 27.9115)
  line L653 (17.9115, 27.9115) -> (11.0885, 27.9115)
  line L654 (4.0885, 16.0885) -> (3.9115, 16.0885)
  line L655 (4.0885, 28.0885) -> (10.9115, 28.0885)
  line L656 (2, 16.0885) -> (3.9115, 16.0885)
  line L657 (4.0885, 27.9115) -> (10.9115, 27.9115)
  line L658 (32.0885, 16.0885) -> (31.9115, 16.0885)
  line L659 (3.9115, 27.9115) -> (2, 27.9115)
  line L660 (18.0885, 15.9115) -> (18.0885, 16.0885)
  line L661 (4.0885, 28.0885) -> (3.9115, 28.0885)
  line L662 (3.9115, 28.0885) -> (3.9115, 27.9115)
  line L663 (25.0885, 16.0885) -> (31.9115, 16.0885)
  line L664 (31.9115, 27.9115) -> (25.0885, 27.9115)
  line L665 (10.9115, 16.0885) -> (11.0885, 16.0885)
  line L666 (31.9115, 28.0885) -> (31.9115, 27.9115)
  line L667 (24.9115, 15.9115) -> (18.0885, 15.9115)
  line L668 (18.0885, 39.9115) -> (18.0885, 40.0885)
  line L669 (24.9115, 16.0885) -> (24.9115, 27.9115)
  line L670 (2, 15.9115) -> (2, 16.0885)
  line L671 (17.9115, 39.9115) -> (18.0885, 39.9115)
  line L672 (3.9115, 16.0885) -> (3.9115, 15.9115)
  line L673 (38.9115, 27.9115) -> (32.0885, 27.9115)
  line L674 (18.0885, 16.0885) -> (17.9115, 16.0885)
  line L675 (3.9115, 16.0885) -> (4.0885, 16.0885)
  line L676 (25.0885, 27.9115) -> (25.0885, 16.0885)
  line L677 (17.9115, 16.0885) -> (17.9115, 15.9115)
  line L678 (3.9115, 28.0885) -> (4.0885, 28.0885)
  line L679 (18.0885, 27.9115) -> (18.0885, 16.0885)
  line L680 (-31.9115, 4.0885) -> (-32.0885, 4.0885)
  line L681 (17.9115, 16.0885) -> (18.0885, 16.0885)
  line L682 (32.0885, 16.0885) -> (31.9115, 16.0885)
  line L683 (3.9115, 28.0885) -> (3.9115, 39.9115)
  line L684 (11.0885, 28.0885) -> (10.9115, 28.0885)
  line L685 (11.0885, 39.9115) -> (11.0885, 28.0885)
  line L686 (24.9115, 39.9115) -> (18.0885, 39.9115)
  line L687 (3.9115, 27.9115) -> (2, 27.9115)
  line L688 (17.9115, 39.9115) -> (11.0885, 39.9115)
  line L689 (18.0885, 28.0885) -> (17.9115, 28.0885)
  line L690 (11.0885, 15.9115) -> (17.9115, 15.9115)
  line L691 (31.9115, 27.9115) -> (25.0885, 27.9115)
  line L692 (25.0885, 27.9115) -> (31.9115, 27.9115)
  line L693 (24.9115, 16.0885) -> (25.0885, 16.0885)
  line L694 (4.0885, 27.9115) -> (4.0885, 28.0885)
  line L695 (17.9115, 15.9115) -> (18.0885, 15.9115)
  line L696 (32.0885, 27.9115) -> (32.0885, 16.0885)
  line L697 (11.0885, 15.9115) -> (11.0885, 16.0885)
  line L698 (11.0885, 27.9115) -> (11.0885, 28.0885)
  line L699 (18.0885, 39.9115) -> (18.0885, 28.0885)
  line L700 (11.0885, 28.0885) -> (10.9115, 28.0885)
  line L701 (11.0885, 16.0885) -> (10.9115, 16.0885)
  line L702 (10.9115, 27.9115) -> (4.0885, 27.9115)
  line L703 (10.9115, 16.0885) -> (10.9115, 15.9115)
  line L704 (10.9115, 28.0885) -> (10.9115, 27.9115)
  line L705 (17.9115, 15.9115) -> (11.0885, 15.9115)
  line L706 (10.9115, 15.9115) -> (11.0885, 15.9115)
  line L707 (11.0885, 16.0885) -> (17.9115, 16.0885)
  line L708 (17.9115, 28.0885) -> (17.9115, 27.9115)
  line L709 (24.9115, 28.0885) -> (24.9115, 27.9115)
  line L710 (17.9115, 39.9115) -> (11.0885, 39.9115)
  line L711 (25.0885, 27.9115) -> (25.0885, 28.0885)
  line L712 (17.9115, 28.0885) -> (18.0885, 28.0885)
  line L713 (25.0885, 28.0885) -> (24.9115, 28.0885)
  line L714 (18.0885, 27.9115) -> (18.0885, 28.0885)
  line L715 (24.9115, 27.9115) -> (18.0885, 27.9115)
  line L716 (18.0885, 28.0885) -> (17.9115, 28.0885)
  line L717 (11.0885, 40.0885) -> (10.9115, 40.0885)
  line L718 (10.9115, 28.0885) -> (10.9115, 39.9115)
  line L719 (4.0885, 28.0885) -> (3.9115, 28.0885)
  line L720 (24.9115, 28.0885) -> (24.9115, 39.9115)
  line L721 (4.0885, 39.9115) -> (4.0885, 28.0885)
  line L722 (10.9115, 39.9115) -> (4.0885, 39.9115)
  line L723 (11.0885, 39.9115) -> (11.0885, 40.0885)
  line L724 (31.9115, 15.9115) -> (32.0885, 15.9115)
  line L725 (2, 28.0885) -> (3.9115, 28.0885)
  line L726 (2, 15.9115) -> (3.9115, 15.9115)
  line L727 (4.0885, 15.9115) -> (4.0885, 4.0885)
  line L728 (32.0885, 15.9115) -> (32.0885, 16.0885)
  line L729 (2, 27.9115) -> (2, 28.0885)
  line L730 (3.9115, 15.9115) -> (4.0885, 15.9115)
  line L731 (24.9115, 15.9115) -> (25.0885, 15.9115)
  line L732 (3.9115, 39.9115) -> (2, 39.9115)
  line L733 (25.0885, 15.9115) -> (31.9115, 15.9115)
  line L734 (32.0885, 28.0885) -> (31.9115, 28.0885)
  line L735 (3.9115, 4.0885) -> (3.9115, 15.9115)
  line L736 (3.9115, 15.9115) -> (2, 15.9115)
  line L737 (4.0885, 39.9115) -> (10.9115, 39.9115)
  line L738 (17.9115, 28.0885) -> (17.9115, 39.9115)
  line L739 (10.9115, 39.9115) -> (11.0885, 39.9115)
  line L740 (4.0885, 4.0885) -> (3.9115, 4.0885)
  line L741 (18.0885, 15.9115) -> (24.9115, 15.9115)
  line L742 (4.0885, 15.9115) -> (10.9115, 15.9115)
  line L743 (11.0885, 39.9115) -> (17.9115, 39.9115)
  line L744 (18.0885, 16.0885) -> (17.9115, 16.0885)
  line L745 (4.0885, 15.9115) -> (4.0885, 16.0885)
  line L746 (18.0885, 16.0885) -> (24.9115, 16.0885)
  line L747 (9.9081, 37.4081) -> (9.9081, 30.5919)
  line L748 (5.0919, -6.5919) -> (9.9081, -6.5919)
  line L749 (-30.9081, 13.4081) -> (-26.0919, 13.4081)
  line L750 (12.0919, 13.4081) -> (16.9081, 13.4081)
  line L751 (-16.9081, 30.5919) -> (-16.9081, 37.4081)
  line L752 (23.9081, -13.4081) -> (19.0919, -13.4081)
  line L753 (9.9081, 30.5919) -> (5.0919, 30.5919)
  line L754 (19.0919, -13.4081) -> (19.0919, -6.5919)
  line L755 (-12.0919, -30.5919) -> (-12.0919, -37.4081)
  line L756 (-10.9115, -15.9115) -> (-11.0885, -15.9115)
  line L757 (9.9081, -13.4081) -> (5.0919, -13.4081)
  line L758 (-12.0919, 37.4081) -> (-12.0919, 30.5919)
  line L759 (-16.9081, -30.5919) -> (-12.0919, -30.5919)
  line L760 (-16.9081, -18.5919) -> (-12.0919, -18.5919)
  line L761 (-16.9081, -25.4081) -> (-16.9081, -18.5919)
  line L762 (16.9081, 30.5919) -> (12.0919, 30.5919)
  line L763 (-12.0919, -25.4081) -> (-16.9081, -25.4081)
  line L764 (-19.0919, -18.5919) -> (-19.0919, -25.4081)
  line L765 (19.0919, -6.5919) -> (23.9081, -6.5919)
  line L766 (-12.0919, -18.5919) -> (-12.0919, -25.4081)
  line L767 (5.0919, -13.4081) -> (5.0919, -6.5919)
  line L768 (26.0919, 25.4081) -> (30.9081, 25.4081)
  line L769 (30.9081, 18.5919) -> (26.0919, 18.5919)
  line L770 (30.9081, 25.4081) -> (30.9081, 18.5919)
  line L771 (26.0919, 18.5919) -> (26.0919, 25.4081)
  line L772 (33.0919, 6.5919) -> (33.0919, 13.4081)
  line L773 (-19.0919, -25.4081) -> (-23.9081, -25.4081)
  line L774 (33.0919, 13.4081) -> (37.9081, 13.4081)
  line L775 (-12.0919, -37.4081) -> (-16.9081, -37.4081)
  line L776 (37.9081, 13.4081) -> (37.9081, 6.5919)
  line L777 (-12.0919, 30.5919) -> (-16.9081, 30.5919)
  line L778 (37.9081, 6.5919) -> (33.0919, 6.5919)
  line L779 (-33.0919, -6.5919) -> (-33.0919, -13.4081)
  line L780 (23.9081, 18.5919) -> (19.0919, 18.5919)
  line L781 (5.0919, -30.5919) -> (9.9081, -30.5919)
  line L782 (-23.9081, -18.5919) -> (-19.0919, -18.5919)
  line L783 (-30.9081, 6.5919) -> (-30.9081, 13.4081)
  line L784 (9.9081, -30.5919) -> (9.9081, -37.4081)
  line L785 (5.0919, -37.4081) -> (5.0919, -30.5919)
  line L786 (9.9081, -37.4081) -> (5.0919, -37.4081)
  line L787 (-37.9081, -6.5919) -> (-33.0919, -6.5919)
  line L788 (19.0919, 6.5919) -> (19.0919, 13.4081)
  line L789 (-16.9081, 37.4081) -> (-12.0919, 37.4081)
  line L790 (12.0919, 18.5919) -> (12.0919, 25.4081)
  line L791 (12.0919, 25.4081) -> (16.9081, 25.4081)
  line L792 (23.9081, 13.4081) -> (23.9081, 6.5919)
  line L793 (26.0919, 6.5919) -> (26.0919, 13.4081)
  line L794 (23.9081, -30.5919) -> (23.9081, -37.4081)
  line L795 (26.0919, -25.4081) -> (26.0919, -18.5919)
  line L796 (30.9081, 6.5919) -> (26.0919, 6.5919)
  line L797 (19.0919, -30.5919) -> (23.9081, -30.5919)
  line L798 (23.9081, -37.4081) -> (19.0919, -37.4081)
  line L799 (30.9081, -18.5919) -> (30.9081, -25.4081)
  line L800 (26.0919, -18.5919) -> (30.9081, -18.5919)
  line L801 (23.9081, 6.5919) -> (19.0919, 6.5919)
  line L802 (16.9081, 18.5919) -> (12.0919, 18.5919)
  line L803 (30.9081, 13.4081) -> (30.9081, 6.5919)
  line L804 (16.9081, 25.4081) -> (16.9081, 18.5919)
  line L805 (26.0919, 13.4081) -> (30.9081, 13.4081)
  line L806 (-16.9081, -37.4081) -> (-16.9081, -30.5919)
  line L807 (19.0919, 13.4081) -> (23.9081, 13.4081)
  line L808 (30.9081, -25.4081) -> (26.0919, -25.4081)
  line L809 (9.9081, -6.5919) -> (9.9081, -13.4081)
  line L810 (19.0919, -37.4081) -> (19.0919, -30.5919)
  line L811 (-23.9081, -25.4081) -> (-23.9081, -18.5919)
  line L812 (9.9081, -25.4081) -> (5.0919, -25.4081)
  line L813 (12.0919, 30.5919) -> (12.0919, 37.4081)
  line L814 (-26.0919, 6.5919) -> (-30.9081, 6.5919)
  line L815 (19.0919, 25.4081) -> (23.9081, 25.4081)
  line L816 (19.0919, 37.4081) -> (23.9081, 37.4081)
  line L817 (5.0919, -25.4081) -> (5.0919, -18.5919)
  line L818 (16.9081, 37.4081) -> (16.9081, 30.5919)
  line L819 (23.9081, 37.4081) -> (23.9081, 30.5919)
  line L820 (-26.0919, 13.4081) -> (-26.0919, 6.5919)
  line L821 (16.9081, 6.5919) -> (12.0919, 6.5919)
  line L822 (23.9081, 30.5919) -> (19.0919, 30.5919)
  line L823 (19.0919, 18.5919) -> (19.0919, 25.4081)
  line L824 (19.0919, 30.5919) -> (19.0919, 37.4081)
  line L825 (-33.0919, -13.4081) -> (-37.9081, -13.4081)
  line L826 (23.9081, 25.4081) -> (23.9081, 18.5919)
  line L827 (9.9081, -18.5919) -> (9.9081, -25.4081)
  line L828 (12.0919, 37.4081) -> (16.9081, 37.4081)
  line L829 (-19.0919, 18.5919) -> (-23.9081, 18.5919)
  line L830 (23.9081, -6.5919) -> (23.9081, -13.4081)
  line L831 (12.0919, 6.5919) -> (12.0919, 13.4081)
  line L832 (5.0919, 30.5919) -> (5.0919, 37.4081)
  line L833 (16.9081, 13.4081) -> (16.9081, 6.5919)
  line L834 (5.0919, 37.4081) -> (9.9081, 37.4081)
  line L835 (-37.9081, -13.4081) -> (-37.9081, -6.5919)
  line L836 (5.0919, -18.5919) -> (9.9081, -18.5919)
  line L837 (-19.0919, 25.4081) -> (-19.0919, 18.5919)
  line L838 (-23.9081, 25.4081) -> (-19.0919, 25.4081)
  line L839 (-23.9081, 18.5919) -> (-23.9081, 25.4081)
  line L840 (-5.0919, -37.4081) -> (-9.9081, -37.4081)
  line L841 (-5.0919, -30.5919) -> (-5.0919, -37.4081)
  line L842 (-9.9081, -30.5919) -> (-5.0919, -30.5919)
  line L843 (-9.9081, -37.4081) -> (-9.9081, -30.5919)
  line L844 (-5.0919, 30.5919) -> (-9.9081, 30.5919)
  line L845 (-5.0919, 37.4081) -> (-5.0919, 30.5919)
  line L846 (-9.9081, 37.4081) -> (-5.0919, 37.4081)
  line L847 (-9.9081, 30.5919) -> (-9.9081, 37.4081)
  line L848 (-5.0919, 18.5919) -> (-9.9081, 18.5919)
  line L849 (-5.0919, 25.4081) -> (-5.0919, 18.5919)
  line L850 (-9.9081, 25.4081) -> (-5.0919, 25.4081)
  line L851 (-9.9081, 18.5919) -> (-9.9081, 25.4081)
  line L852 (-26.0919, -25.4081) -> (-30.9081, -25.4081)
  line L853 (-26.0919, -18.5919) -> (-26.0919, -25.4081)
  line L854 (-30.9081, -18.5919) -> (-26.0919, -18.5919)
  line L855 (-30.9081, -25.4081) -> (-30.9081, -18.5919)
  line L856 (-12.0919, 18.5919) -> (-16.9081, 18.5919)
  line L857 (-12.0919, 25.4081) -> (-12.0919, 18.5919)
  line L858 (-16.9081, 25.4081) -> (-12.0919, 25.4081)
  line L859 (-16.9081, 18.5919) -> (-16.9081, 25.4081)
  line L860 (16.9081, -25.4081) -> (12.0919, -25.4081)
  line L861 (16.9081, -18.5919) -> (16.9081, -25.4081)
  line L862 (12.0919, -18.5919) -> (16.9081, -18.5919)
  line L863 (12.0919, -25.4081) -> (12.0919, -18.5919)
  line L864 (-19.0919, -37.4081) -> (-23.9081, -37.4081)
  line L865 (-19.0919, -30.5919) -> (-19.0919, -37.4081)
  line L866 (-23.9081, -30.5919) -> (-19.0919, -30.5919)
  line L867 (-23.9081, -37.4081) -> (-23.9081, -30.5919)
  line L868 (-26.0919, 18.5919) -> (-30.9081, 18.5919)
  line L869 (-26.0919, 25.4081) -> (-26.0919, 18.5919)
  line L870 (-30.9081, 25.4081) -> (-26.0919, 25.4081)
  line L871 (-30.9081, 18.5919) -> (-30.9081, 25.4081)
  line L872 (23.9081, -25.4081) -> (19.0919, -25.4081)
  line L873 (23.9081, -18.5919) -> (23.9081, -25.4081)
  line L874 (19.0919, -18.5919) -> (23.9081, -18.5919)
  line L875 (19.0919, -25.4081) -> (19.0919, -18.5919)
  line L876 (9.9081, 18.5919) -> (5.0919, 18.5919)
  line L877 (9.9081, 25.4081) -> (9.9081, 18.5919)
  line L878 (5.0919, 25.4081) -> (9.9081, 25.4081)
  line L879 (5.0919, 18.5919) -> (5.0919, 25.4081)
  line L880 (-19.0919, 6.5919) -> (-23.9081, 6.5919)
  line L881 (-19.0919, 13.4081) -> (-19.0919, 6.5919)
  line L882 (-23.9081, 13.4081) -> (-19.0919, 13.4081)
  line L883 (-23.9081, 6.5919) -> (-23.9081, 13.4081)
  line L884 (0.1, -49) -> (-0.1, -49)
  line L885 (0.1, 49) -> (0.1, -49)
  line L886 (-0.1, 49) -> (0.1, 49)
  line L887 (-0.1, -49) -> (-0.1, 49)
  line L888 (49, -0.1) -> (-49, -0.1)
  line L889 (49, 0.1) -> (49, -0.1)
  line L890 (-49, 0.1) -> (49, 0.1)
  line L891 (-49, -0.1) -> (-49, 0.1)
  line L892 (37.9081, -13.4081) -> (33.0919, -13.4081)
  line L893 (37.9081, -6.5919) -> (37.9081, -13.4081)
  line L894 (33.0919, -6.5919) -> (37.9081, -6.5919)
  line L895 (33.0919, -13.4081) -> (33.0919, -6.5919)
  line L896 (-5.0919, 6.5919) -> (-9.9081, 6.5919)
  line L897 (-5.0919, 13.4081) -> (-5.0919, 6.5919)
  line L898 (-9.9081, 13.4081) -> (-5.0919, 13.4081)
  line L899 (-9.9081, 6.5919) -> (-9.9081, 13.4081)
  line L900 (-19.0919, -13.4081) -> (-23.9081, -13.4081)
  line L901 (-19.0919, -6.5919) -> (-19.0919, -13.4081)
  line L902 (-23.9081, -6.5919) -> (-19.0919, -6.5919)
  line L903 (-23.9081, -13.4081) -> (-23.9081, -6.5919)
  line L904 (9.9081, 6.5919) -> (5.0919, 6.5919)
  line L905 (9.9081, 13.4081) -> (9.9081, 6.5919)
  line L906 (5.0919, 13.4081) -> (9.9081, 13.4081)
  line L907 (5.0919, 6.5919) -> (5.0919, 13.4081)
  line L908 (-19.0919, 30.5919) -> (-23.9081, 30.5919)
  line L909 (-19.0919, 37.4081) -> (-19.0919, 30.5919)
  line L910 (-23.9081, 37.4081) -> (-19.0919, 37.4081)
  line L911 (-23.9081, 30.5919) -> (-23.9081, 37.4081)
  line L912 (-12.0919, 6.5919) -> (-16.9081, 6.5919)
  line L913 (-12.0919, 13.4081) -> (-12.0919, 6.5919)
  line L914 (-16.9081, 13.4081) -> (-12.0919, 13.4081)
  line L915 (-16.9081, 6.5919) -> (-16.9081, 13.4081)
  line L916 (-12.0919, -13.4081) -> (-16.9081, -13.4081)
  line L917 (-12.0919, -6.5919) -> (-12.0919, -13.4081)
  line L918 (-16.9081, -6.5919) -> (-12.0919, -6.5919)
  line L919 (-16.9081, -13.4081) -> (-16.9081, -6.5919)
  line L920 (-5.0919, -13.4081) -> (-9.9081, -13.4081)
  line L921 (-5.0919, -6.5919) -> (-5.0919, -13.4081)
  line L922 (-9.9081, -6.5919) -> (-5.0919, -6.5919)
  line L923 (-9.9081, -13.4081) -> (-9.9081, -6.5919)
  line L924 (-5.0919, -25.4081) -> (-9.9081, -25.4081)
  line L925 (-5.0919, -18.5919) -> (-5.0919, -25.4081)
  line L926 (-9.9081, -18.5919) -> (-5.0919, -18.5919)
  line L927 (-9.9081, -25.4081) -> (-9.9081, -18.5919)
  line L928 (16.9081, -37.4081) -> (12.0919, -37.4081)
  line L929 (16.9081, -30.5919) -> (16.9081, -37.4081)
  line L930 (12.0919, -30.5919) -> (16.9081, -30.5919)
  line L931 (12.0919, -37.4081) -> (12.0919, -30.5919)
  line L932 (-26.0919, -13.4081) -> (-30.9081, -13.4081)
  line L933 (-26.0919, -6.5919) -> (-26.0919, -13.4081)
  line L934 (-30.9081, -6.5919) -> (-26.0919, -6.5919)
  line L935 (-30.9081, -13.4081) -> (-30.9081, -6.5919)
  line L936 (16.9081, -13.4081) -> (12.0919, -13.4081)
  line L937 (16.9081, -6.5919) -> (16.9081, -13.4081)
  line L938 (12.0919, -6.5919) -> (16.9081, -6.5919)
  line L939 (12.0919, -13.4081) -> (12.0919, -6.5919)
  line L940 (-33.0919, 6.5919) -> (-37.9081, 6.5919)
  line L941 (-33.0919, 13.4081) -> (-33.0919, 6.5919)
  line L942 (-37.9081, 13.4081) -> (-33.0919, 13.4081)
  line L943 (-37.9081, 6.5919) -> (-37.9081, 13.4081)
  line L944 (30.9081, -13.4081) -> (26.0919, -13.4081)
  line L945 (30.9081, -6.5919) -> (30.9081, -13.4081)
  line L946 (26.0919, -6.5919) -> (30.9081, -6.5919)